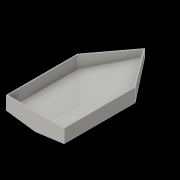
# Autodesk Inventor part: Generalcraftshape1
Saved by Autodesk Inventor 2016 (Build 200138000, 138)
## iProperties
Created: 2019-01-02
Part Number: Generalcraftshape1
Material: Generic
Document SubType Name: Modeling
Designer: LinJie
Density: 1 g/cm^3
Appearance: Default
Author: LinJie
Autodesk Inventor part; units mm, degrees
ref_plane "YZ Plane" through (0, 0, 0) normal (1, 0, 0) x (0, 1, 0)
ref_plane "XZ Plane" through (0, 0, 0) normal (0, 1, 0) x (-1, 0, 0)
ref_plane "XY Plane" through (0, 0, 0) normal (0, 0, 1) x (1, 0, 0)
sketch "Sketch1" plane through (0, 0, 0) normal (0, 1, 0) x (-1, 0, 0)
  line L0 (150, 70) -> (-150, 70)
  line L1 (-150, 70) -> (-150, 0)
  line L2 (-150, 0) -> (150, 0)
  line L3 (150, 0) -> (150, 70)
  line L4 (150, 0) -> (0, -20)
  line L5 (0, -20) -> (-150, 0)
  point P0 (0, 0)
  point P1 (0, 0)
  dimension "d0" = 300
  dimension "d1" = 70
  dimension "d2" = 20
  constraints: 12 end point, 2 parallel, 1 coincident, 1 equal length, 1 horizontal, 1 midpoint, 1 perpendicular
  measures "d0" distance of L1.end L2.end
  measures "d1" distance of L0.end L1.end
  measures "d2" distance of L4.end point (0, 0)
extrude "Extrusion1" add sketch "Sketch1" along normal blind 600
sketch "Sketch2" plane through (-150, 0, 70) normal (0, 0, 1) x (1, 0, 0)
  line L0 (0, 0) -> (300, 0) projected
  line L1 (300, 0) -> (300, 600) projected
  line L2 (0, 600) -> (300, 600) projected
  line L3 (0, 0) -> (0, 600) projected
  ellipse E0 centre (150, 370) end of major axis (0, 370) minor radius 200
  line L4 (0, 370) -> (150, 570)
  line L5 (150, 570) -> (300, 370)
  point P0 (150, 0)
  point P1 (150, 600)
  dimension "d7" = 200
  dimension "d5" = 370
  constraints: 4 end point, 2 point on line, 1 equal length, 1 midpoint, 1 vertical, 1 vertical alignment, 5 other
  measures "d5" distance from line of L0 point (150, 370)
extrude "Extrusion2" cut sketch "Sketch2" against normal through all contours L3 L2 L1 E0 | E0 L4 | L5 E0
sketch "Sketch3" plane through (-150, 0, 0) normal (-1, 0, 0) x (0, 0, 1)
  line L0 (70, 570) -> (-20, 570) projected
  line L1 (-20, 0) -> (-20, 570) projected
  line L2 (30, 570) -> (-20, 236.6667)
  point P0 (0, 0)
  point P1 (0, 370)
  dimension "d11" = 40
  constraints: 3 point on line, 2 end point
  measures "d11" distance of L0.start L2.start
extrude "Extrusion3" cut sketch "Sketch3" against normal through all
shell "Shell2" thickness 4 removed faces 1 at (50, 246.6667, 70)
body "Solid1"
